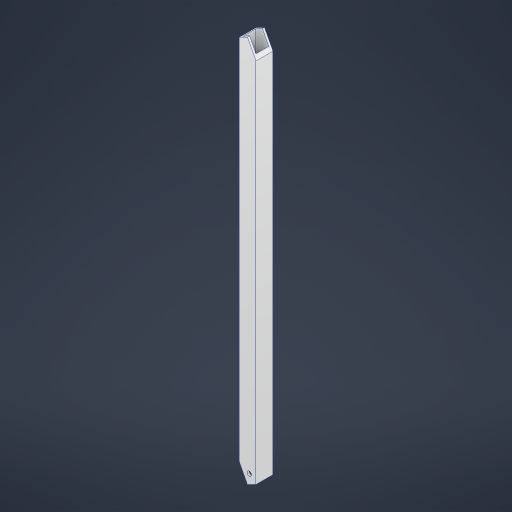
# Autodesk Inventor part: STRU_013_BilletCrossbar2_Angled
Saved by Autodesk Inventor 2024.2 (Build 282272000, 272)
## iProperties
Created: 2024-07-25
Part Number: STRU_013_BilletCrossbar2_Angled
Material: Aluminum 6061
Document SubType Name: Modeling
Designer: Bryan
Density: 2.7 g/cm^3
Appearance: Aluminum - Flat
Mass: 425.32 g
Surface Area: 1002.41 cm^2
Volume: 157.526 cm^3
Author: Bryan
Autodesk Inventor part; units mm, degrees
ref_plane "YZ Plane" through (0, 0, 0) normal (1, 0, 0) x (0, 1, 0)
ref_plane "XZ Plane" through (0, 0, 0) normal (0, 1, 0) x (-1, 0, 0)
ref_plane "XY Plane" through (0, 0, 0) normal (0, 0, 1) x (1, 0, 0)
sketch "Sketch1" plane through (0, 0, 0) normal (0, 1, 0) x (-1, 0, 0)
  line L0 (-12.7, -12.7) -> (12.7, -12.7)
  line L1 (12.7, -12.7) -> (12.7, 12.7)
  line L2 (12.7, 12.7) -> (-12.7, 12.7)
  line L3 (-12.7, 12.7) -> (-12.7, -12.7)
  line L4 (-12.7, -12.7) -> (12.7, 12.7) construction
  line L5 (12.7, -12.7) -> (-12.7, 12.7) construction
  line L6 (9.525, 9.525) -> (9.525, -9.525)
  line L7 (9.525, -9.525) -> (-9.525, -9.525)
  line L8 (-9.525, -9.525) -> (-9.525, 9.525)
  line L9 (-9.525, 9.525) -> (9.525, 9.525)
  point P0 (0, 0)
  dimension "d0" = 25.4
  dimension "d1" = 25.4
  dimension "d2" = 3.175
  constraints: 20 end point, 4 parallel, 2 midpoint, 2 perpendicular, 1 horizontal, 3 other
  measures "d0" distance of L2.end L1.end
  measures "d1" distance of L1.end L0.end
  measures "d2" distance between parallel lines of L1 L6
extrude "Extrusion1" add sketch "Sketch1" along normal blind 579.374
sketch "Sketch4" plane through (-12.7, 0, 12.7) normal (0, 0, 1) x (1, 0, 0)
  line L0 (249.4631, 122.7685) -> (12.7, 579.374)
  line L1 (12.7, 579.374) -> (-224.0631, 456.6055)
  line L2 (-224.0631, 456.6055) -> (12.7, 0)
  line L3 (12.7, 0) -> (249.4631, 122.7685)
  line L4 (0, 0) -> (25.4, 0) projected
  line L5 (0, 579.374) -> (25.4, 579.374) projected
  line L6 (0, 0) -> (25.4, 0) projected
  line L7 (25.4, 0) -> (25.4, 579.374) projected
  line L8 (0, 579.374) -> (25.4, 579.374) projected
  line L9 (0, 0) -> (0, 579.374) projected
  point P0 (0, 24.4924)
  point P1 (25.4, 6.5853)
  point P2 (0, 572.7887)
  point P3 (25.4, 554.8816)
  dimension "d13" = 266.7
  constraints: 8 end point, 2 midpoint, 2 parallel, 1 perpendicular
  measures "d13" distance of L0.end L1.end
extrude "Extrusion4" cut sketch "Sketch4" against normal blind 370.4968 contours L0 L5 L7 | L7 L4 L3 | L1 L9 L5 | L4 L9 L2
sketch "Sketch6" plane through (12.7, 6.5853, 12.7) normal (0, 0, 1) x (1, 0, 0)
  line L0 (-24.3922, 15.9636) -> (-46.9411, 4.2713) construction
  line L1 (-46.9411, 4.2713) -> (-35.2489, -18.2776) construction
  line L2 (-35.2489, -18.2776) -> (-12.7, -6.5853) construction
  line L3 (-12.7, -6.5853) -> (-25.4, 17.9071) construction
  line L4 (-25.4, 17.9071) -> (-12.7, -6.5853) construction
  line L5 (-46.9411, 4.2713) -> (-12.7, -6.5853) construction
  circle A0 centre (-29.8206, -1.157) radius 3.2512 construction
  circle A1 centre (-10.0903, 9.0737) radius 3.2512
  line L6 (-41.095, -7.0031) -> (-4.5992, 11.921) construction
  dimension "d21" = 25.4
  dimension "d22" = 25.4
  dimension "d23" = 6.5024
  dimension "d24" = 6.5024
  dimension "d25" = 22.225
  constraints: 12 end point, 3 point on line, 2 centre point, 2 midpoint, 2 parallel, 2 perpendicular
  measures "d21" distance of L0.start L0.end
  measures "d22" distance of L1.end L0.end
  measures "d23" diameter of A0
  measures "d24" diameter of A1
  measures "d25" distance of A0.centre A1.centre
extrude "Extrusion6" cut sketch "Sketch6" against normal blind 25.4
body "Solid1"
